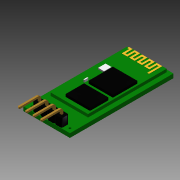
# Autodesk Inventor part: JY-MCU Bluetooth Board
Saved by Autodesk Inventor 2014 (Build 180170000, 170)
## iProperties
Created: 2014-02-20
Part Number: JY-MCU Bluetooth Board
Material: PAEK Plastic
Document SubType Name: Modeling
Designer: Spooner
Density: 1.32 g/cm^3
Appearance: Dark Green
Author: Spooner
Autodesk Inventor part; units mm, degrees
ref_plane "YZ Plane" through (0, 0, 0) normal (1, 0, 0) x (0, 1, 0)
ref_plane "XZ Plane" through (0, 0, 0) normal (0, 1, 0) x (-1, 0, 0)
ref_plane "XY Plane" through (0, 0, 0) normal (0, 0, 1) x (1, 0, 0)
sketch "Sketch1" plane through (0, 0, 0) normal (0, 1, 0) x (-1, 0, 0)
  line L0 (0, 0) -> (15.9512, 0)
  line L1 (15.9512, 0) -> (15.9512, 35.56)
  line L2 (15.9512, 35.56) -> (0, 35.56)
  line L3 (0, 35.56) -> (0, 0)
  dimension "d0" = 15.9512
  dimension "d1" = 35.56
  constraints: 8 end point, 2 parallel, 1 horizontal, 1 perpendicular
  measures "d0" distance of L0.start L0.end
  measures "d1" distance of L2.end L0.start
extrude "Extrusion1" add sketch "Sketch1" along normal blind 1.397
sketch "Sketch2" plane through (0, 1.397, 0) normal (0, 1, 0) x (1, 0, 0)
  line L0 (0, 0) -> (-15.9512, 0) projected
  line L1 (-15.9512, 0) -> (-15.9512, -35.56) projected
  line L2 (0, -35.56) -> (0, 0) projected
  line L3 (-14.3891, -0.762) -> (-1.5621, -0.762)
  line L4 (-1.5621, -0.762) -> (-1.5621, -27.7622)
  line L5 (-1.5621, -27.7622) -> (-14.3891, -27.7622)
  line L6 (-14.3891, -27.7622) -> (-14.3891, -0.762)
  dimension "d4" = 12.827
  dimension "d5" = 1.5621
  dimension "d6" = 1.5621
  dimension "d7" = 27.0002
  dimension "d8" = 0.762
  constraints: 8 end point, 2 parallel, 1 horizontal, 1 perpendicular
  measures "d4" distance of L4.end L5.end
  measures "d5" distance between parallel lines of L2 L4
  measures "d6" distance between parallel lines of L1 L6
  measures "d7" distance of L5.end L3.start
  measures "d8" distance between parallel lines of L0 L3
extrude "Extrusion2" add sketch "Sketch2" along normal blind 1.016
sketch "Sketch3" plane through (0, 2.413, 0) normal (0, 1, 0) x (1, 0, 0)
  line L0 (-1.5621, -0.762) -> (-14.3891, -0.762) projected
  line L1 (-1.5621, -27.7622) -> (-1.5621, -0.762) projected
  line L2 (-10.5537, -10.2362) -> (-2.1717, -10.2362)
  line L3 (-2.1717, -10.2362) -> (-2.1717, -18.6182)
  line L4 (-2.1717, -18.6182) -> (-10.5537, -18.6182)
  line L5 (-10.5537, -18.6182) -> (-10.5537, -10.2362)
  line L6 (-10.5537, -26.4922) -> (-2.1717, -26.4922)
  line L7 (-2.1717, -26.4922) -> (-2.1717, -20.1422)
  line L8 (-2.1717, -20.1422) -> (-10.5537, -20.1422)
  line L9 (-10.5537, -20.1422) -> (-10.5537, -26.4922)
  point P0 (0, 0)
  dimension "d11" = 8.382
  dimension "d12" = 6.35
  dimension "d13" = 1.524
  dimension "d14" = 9.4742
  dimension "d15" = 0.6096
  constraints: 16 end point, 4 parallel, 3 perpendicular, 2 horizontal, 2 vertical alignment
  measures "d11" distance of L2.end L3.end
  measures "d12" distance of L6.end L7.end
  measures "d13" distance between parallel lines of L8 L4
  measures "d14" distance between parallel lines of L0 L2
  measures "d15" distance between parallel lines of L1 L7
extrude "Extrusion3" add sketch "Sketch3" along normal blind 0.8382
sketch "Sketch4" plane through (0, 1.397, 0) normal (0, 1, 0) x (1, 0, 0)
  line L0 (-15.9512, 0) -> (-15.9512, -35.56) projected
  line L1 (-15.9512, -35.56) -> (0, -35.56) projected
  line L2 (0, -35.56) -> (0, 0) projected
  circle A0 centre (-14.4653, -34.0741) radius 0.3683
  circle A1 centre (-1.4859, -34.0741) radius 0.3683
  dimension "d18" = 0.7366
  dimension "d19" = 1.1176
  dimension "d20" = 1.1176
  dimension "d21" = 1.1176
  constraints: 2 centre point, 1 equal radius, 1 horizontal alignment
  measures "d18" diameter of A0
  measures "d19" distance edge to line of A0 L0
  measures "d20" distance edge to line of A1 L2
  measures "d21" distance edge to line of A0 L1
extrude "Extrusion4" cut sketch "Sketch4" against normal through all
sketch "Sketch5" plane through (0, 1.397, 0) normal (0, 1, 0) x (1, 0, 0)
  line L0 (-15.9512, 0) -> (-15.9512, -35.56) projected
  line L1 (-15.9512, -35.56) -> (0, -35.56) projected
  line L2 (-13.0302, -32.9946) -> (-10.5664, -32.9946)
  line L3 (-10.5664, -32.9946) -> (-10.5664, -35.4584)
  line L4 (-10.5664, -35.4584) -> (-13.0302, -35.4584)
  line L5 (-13.0302, -35.4584) -> (-13.0302, -32.9946)
  dimension "d24" = 2.4638
  dimension "d25" = 0.1016
  dimension "d26" = 2.921
  constraints: 8 end point, 2 parallel, 2 perpendicular, 1 horizontal
  measures "d24" distance of L4.end L2.start
  measures "d25" distance between parallel lines of L1 L4
  measures "d26" distance between parallel lines of L0 L5
extrude "Extrusion5" add sketch "Sketch5" along normal blind 2.8702
fillet "Fillet1" radius 0.508 4 edges at (-10.5664, 2.8321, 35.4584) (-13.0302, 2.8321, 35.4584) (-10.5664, 2.8321, 32.9946) (-13.0302, 2.8321, 32.9946)
ref_plane "Work Plane1" through (-12.2682, 1.397, 33.5026) normal (-1, 0, 0) x (0, 0, 1)
sketch "Sketch6" plane through (-12.2682, 1.397, 33.5026) normal (-1, 0, 0) x (0, 0, 1)
  line L0 (0.254, 2.8702) -> (0.254, 3.6322)
  arc A0 (1.397, 4.7752) -> (0.254, 3.6322) centre (1.397, 3.6322) ccw
  line L1 (1.397, 4.7752) -> (7.874, 4.7752)
  line L2 (7.874, 4.7752) -> (7.874, 4.1402)
  line L3 (7.874, 4.1402) -> (1.397, 4.1402)
  arc A1 (1.397, 4.1402) -> (0.889, 3.6322) centre (1.397, 3.6322) ccw
  line L4 (0.889, 3.6322) -> (0.889, 2.8702)
  line L5 (0.889, 2.8702) -> (0.254, 2.8702)
  line L6 (0, 2.8702) -> (0, 0) projected
  line L7 (1.4478, 2.8702) -> (0, 2.8702) projected
  line L8 (1.4478, 0) -> (1.4478, 2.8702) projected
  line L9 (0, 0) -> (1.4478, 0) projected
  line L10 (-0.508, 2.8702) -> (0, 2.8702) projected
  line L11 (1.4478, 2.8702) -> (1.9558, 2.8702) projected
  point P0 (-33.5026, -1.397)
  dimension "d34" = 0.635
  dimension "d35" = 0.635
  dimension "d36" = 0.635
  dimension "d37" = 1.905
  dimension "d38" = 7.62
  dimension "d39" = 0.762
  dimension "d40" = 1.143
  constraints: 12 end point, 4 perpendicular, 4 point on circle, 4 tangent, 2 centre point, 1 parallel, 1 point on line, 1 vertical
  measures "d34" distance between parallel lines of L3 L1
  measures "d35" distance between parallel lines of L0 L4
  measures "d36" radial gap between concentric circles of A0 A1
  measures "d37" distance from line of L7.start L1
  measures "d38" distance between parallel lines of L0 L2
  measures "d39" distance from line of L10.start L0
  measures "d40" radius of A0
extrude "Extrusion6" add sketch "Sketch6" against normal blind 0.635 contours L0 A0 L1 L2 L3 A1 L4 L5
chamfer "Chamfer1" distance 0.254 angle 45 4 edges at (-11.9507, 6.1722, 41.3766) (-11.6332, 5.8547, 41.3766) (-11.9507, 5.5372, 41.3766) (-12.2682, 5.8547, 41.3766)
sketch "Sketch7" plane through (0, 0, 0) normal (0, -1, 0) x (1, 0, 0)
  line L0 (-12.2682, 33.7566) -> (-11.6332, 33.7566) projected
  line L1 (-12.2682, 34.3916) -> (-12.2682, 33.7566) projected
  line L2 (-11.6332, 34.3916) -> (-12.2682, 34.3916) projected
  line L3 (-11.6332, 33.7566) -> (-11.6332, 34.3916) projected
  circle A0 centre (-11.9507, 34.0741) radius 0.3175
  constraints: 3 tangent, 1 centre point
extrude "Extrusion7" add sketch "Sketch7" along normal blind 0.508 contours A0
chamfer "Chamfer2" distance 0.254 angle 45 1 edges at (-12.2682, -0.508, 34.0741)
fillet "Fillet2" radius 0.254 1 edges at (-12.2682, 0, 34.0741)
pattern_linear "Rectangular Pattern2" count 4 spacing 2.54 along (1, 0, 0) of "Extrusion5", "Fillet1", "Extrusion6", "Chamfer1", "Extrusion7", "Chamfer2", "Fillet2"
sketch "Sketch8" plane through (0, 2.413, 0) normal (0, 1, 0) x (1, 0, 0)
  line L0 (-2.1717, -18.6182) -> (-10.5537, -18.6182) projected
  line L1 (-10.5537, -18.6182) -> (-10.5537, -10.2362) projected
  line L2 (-11.9253, -17.653) -> (-11.5443, -17.653)
  line L3 (-11.5443, -17.653) -> (-11.5443, -18.9992)
  line L4 (-11.5443, -18.9992) -> (-11.9253, -18.9992)
  line L5 (-11.9253, -18.9992) -> (-11.9253, -17.653)
  point P0 (0, 0)
  dimension "d55" = 1.3462
  dimension "d56" = 0.381
  dimension "d57" = 0.9906
  dimension "d58" = 0.381
  constraints: 8 end point, 2 parallel, 1 horizontal, 1 perpendicular
  measures "d55" distance of L4.end L2.start
  measures "d56" distance of L3.end L4.end
  measures "d57" distance between parallel lines of L3 L1
  measures "d58" distance between parallel lines of L0 L4
extrude "Extrusion8" add sketch "Sketch8" along normal blind 0.762
sketch "Sketch9" plane through (0, 2.413, 0) normal (0, 1, 0) x (1, 0, 0)
  line L0 (-1.5621, -0.762) -> (-14.3891, -0.762) projected
  line L1 (-14.3891, -0.762) -> (-14.3891, -27.7622) projected
  line L2 (-1.5621, -27.7622) -> (-1.5621, -0.762) projected
  line L3 (-14.3891, -0.8636) -> (-13.1191, -0.8636)
  line L4 (-13.1191, -0.8636) -> (-13.1191, -3.4036)
  line L5 (-13.1191, -3.4036) -> (-12.4841, -3.4036)
  line L6 (-12.4841, -3.4036) -> (-12.4841, -0.8636)
  line L7 (-12.4841, -0.8636) -> (-10.5791, -0.8636)
  line L8 (-10.5791, -0.8636) -> (-10.5791, -3.4036)
  line L9 (-10.5791, -3.4036) -> (-9.9441, -3.4036)
  line L10 (-9.9441, -3.4036) -> (-9.9441, -0.8636)
  line L11 (-9.9441, -0.8636) -> (-8.0391, -0.8636)
  line L12 (-8.0391, -0.8636) -> (-8.0391, -3.4036)
  line L13 (-8.0391, -3.4036) -> (-7.4041, -3.4036)
  line L14 (-7.4041, -3.4036) -> (-7.4041, -0.8636)
  line L15 (-7.4041, -0.8636) -> (-5.4991, -0.8636)
  line L16 (-5.4991, -0.8636) -> (-5.4991, -3.4036)
  line L17 (-5.4991, -3.4036) -> (-4.8641, -3.4036)
  line L18 (-4.8641, -3.4036) -> (-4.8641, -0.8636)
  line L19 (-4.8641, -0.8636) -> (-2.9591, -0.8636)
  line L20 (-2.9591, -0.8636) -> (-2.9591, -5.4356)
  line L21 (-2.9591, -5.4356) -> (-3.5941, -5.4356)
  line L22 (-3.5941, -5.4356) -> (-3.5941, -1.4986)
  line L23 (-3.5941, -1.4986) -> (-4.2291, -1.4986)
  line L24 (-4.2291, -1.4986) -> (-4.2291, -4.0386)
  line L25 (-4.2291, -4.0386) -> (-6.1341, -4.0386)
  line L26 (-6.1341, -4.0386) -> (-6.1341, -1.4986)
  line L27 (-6.1341, -1.4986) -> (-6.7691, -1.4986)
  line L28 (-6.7691, -1.4986) -> (-6.7691, -4.0386)
  line L29 (-6.7691, -4.0386) -> (-8.6741, -4.0386)
  line L30 (-8.6741, -4.0386) -> (-8.6741, -1.4986)
  line L31 (-8.6741, -1.4986) -> (-9.3091, -1.4986)
  line L32 (-9.3091, -1.4986) -> (-9.3091, -4.0386)
  line L33 (-9.3091, -4.0386) -> (-11.2141, -4.0386)
  line L34 (-11.2141, -4.0386) -> (-11.2141, -1.4986)
  line L35 (-11.2141, -1.4986) -> (-11.8491, -1.4986)
  line L36 (-11.8491, -1.4986) -> (-11.8491, -4.0386)
  line L37 (-11.8491, -4.0386) -> (-13.7541, -4.0386)
  line L38 (-13.7541, -4.0386) -> (-13.7541, -1.4986)
  line L39 (-13.7541, -1.4986) -> (-14.3891, -1.4986)
  line L40 (-14.3891, -0.8636) -> (-14.3891, -1.4986)
  point P0 (0, 0)
  dimension "d61" = 0.635
  dimension "d62" = 0.635
  dimension "d63" = 0.635
  dimension "d64" = 0.635
  dimension "d65" = 0.635
  dimension "d66" = 0.635
  dimension "d67" = 0.635
  dimension "d68" = 0.635
  dimension "d69" = 0.635
  dimension "d70" = 0.635
  dimension "d71" = 0.635
  dimension "d72" = 0.635
  dimension "d73" = 0.635
  dimension "d74" = 0.635
  dimension "d75" = 0.635
  dimension "d76" = 0.635
  dimension "d77" = 0.635
  dimension "d78" = 0.635
  dimension "d79" = 0.635
  dimension "d80" = 0.635
  dimension "d81" = 1.397
  dimension "d82" = 3.175
  dimension "d83" = 0.1016
  dimension "d84" = 4.572
  constraints: 76 end point, 21 parallel, 14 horizontal alignment, 13 perpendicular, 4 collinear, 2 point on line
  measures "d61" distance between parallel lines of L3 L39
  measures "d62" distance between parallel lines of L38 L4
  measures "d63" distance between parallel lines of L37 L5
  measures "d64" distance between parallel lines of L36 L6
  measures "d65" distance between parallel lines of L8 L34
  measures "d66" distance between parallel lines of L32 L10
  measures "d67" distance between parallel lines of L12 L30
  measures "d68" distance between parallel lines of L28 L14
  measures "d69" distance between parallel lines of L26 L16
  measures "d70" distance between parallel lines of L24 L18
  measures "d71" distance between parallel lines of L20 L22
  measures "d72" distance between parallel lines of L6 L4
  measures "d73" distance between parallel lines of L36 L34
  measures "d74" distance between parallel lines of L10 L8
  measures "d75" distance between parallel lines of L30 L32
  measures "d76" distance between parallel lines of L14 L12
  measures "d77" distance between parallel lines of L26 L28
  measures "d78" distance between parallel lines of L18 L16
  measures "d79" distance between parallel lines of L22 L24
  measures "d80" distance between parallel lines of L1 L38
  measures "d81" distance between parallel lines of L2 L20
  measures "d82" distance between parallel lines of L37 L3
  measures "d83" distance between parallel lines of L0 L7
  measures "d84" distance of L19.end L20.end
extrude "Extrusion9" add sketch "Sketch9" along normal blind 0.1016
sketch "Sketch10" plane through (0, 2.413, 0) normal (0, 1, 0) x (1, 0, 0)
  line L0 (-10.5537, -18.6182) -> (-10.5537, -10.2362) projected
  line L1 (-13.0937, -10.2362) -> (-11.0617, -10.2362)
  line L2 (-11.0617, -10.2362) -> (-11.0617, -12.7762)
  line L3 (-11.0617, -12.7762) -> (-13.0937, -12.7762)
  line L4 (-13.0937, -12.7762) -> (-13.0937, -10.2362)
  point P0 (0, 0)
  dimension "d87" = 2.54
  dimension "d88" = 2.032
  dimension "d89" = 0.508
  constraints: 8 end point, 2 parallel, 1 horizontal, 1 horizontal alignment, 1 perpendicular
  measures "d87" distance of L3.end L1.start
  measures "d88" distance of L1.start L1.end
  measures "d89" distance between parallel lines of L0 L2
extrude "Extrusion10" add sketch "Sketch10" along normal blind 0.508
ref_plane "Work Plane2" through (-9.7282, 1.397, 33.5026) normal (-1, 0, 0) x (0, 0, 1)
ref_plane "Work Plane3" through (-7.1882, 1.397, 33.5026) normal (-1, 0, 0) x (0, 0, 1)
ref_plane "Work Plane4" through (-4.6482, 1.397, 33.5026) normal (-1, 0, 0) x (0, 0, 1)
equation "\"d5\" = d6"
equation "\"d20\" = d19"
equation "\"d21\" = d19"
equation "\"d35\" = d34"
equation "\"d36\" = d34"
equation "\"d62\" = d61"
equation "\"d63\" = d62"
equation "\"d64\" = d62"
equation "\"d65\" = d62"
equation "\"d66\" = d65"
equation "\"d67\" = d65"
equation "\"d68\" = d67"
equation "\"d69\" = d68"
equation "\"d70\" = d69"
equation "\"d71\" = d70"
equation "\"d72\" = d62"
equation "\"d73\" = d64"
equation "\"d74\" = d64"
equation "\"d75\" = d74"
equation "\"d76\" = d75"
equation "\"d77\" = d76"
equation "\"d78\" = d77"
equation "\"d79\" = d78"
body "Solid1"
